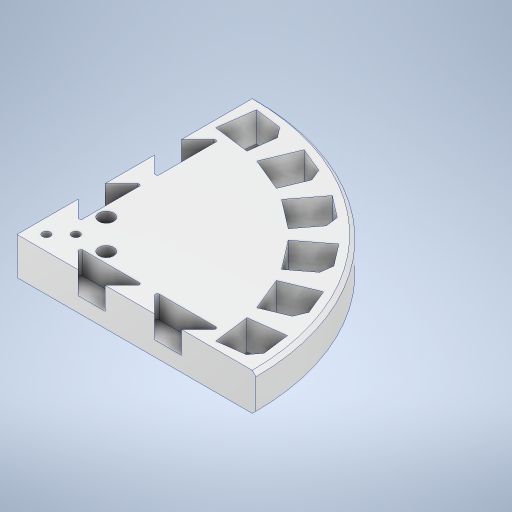
# Autodesk Inventor part: IPT_Quarter_Sample_Tray
Saved by Autodesk Inventor 2024 (Build 280153000, 153)
## iProperties
Created: 2023-10-26
Part Number: IPT_Quarter_Sample_Tray
Material: Generic
Document SubType Name: Modeling
Designer: Besher
Density: 1 g/cm^3
Appearance: Aluminum - Flat
Author: Besher
Autodesk Inventor part; units mm, degrees
ref_plane "YZ Plane" through (0, 0, 0) normal (1, 0, 0) x (0, 1, 0)
ref_plane "XZ Plane" through (0, 0, 0) normal (0, 1, 0) x (-1, 0, 0)
sketch "Sketch1" plane through (0, 0, 0) normal (0, 1, 0) x (-1, 0, 0)
  circle A0 centre (0, 0) radius 203.2
  dimension "d0" = 406.4
  constraints: 1 centre point
  measures "d0" diameter of A0
extrude "Extrusion1" add sketch "Sketch1" along normal blind 38.1
sketch "Sketch3" plane through (0, 38.1, 0) normal (0, 1, 0) x (1, 0, 0)
  circle A0 centre (0, 0) radius 203.2 projected
  line L0 (0, 203.2) -> (0, 177.8)
  line L1 (-15.367, 193.167) -> (15.367, 193.167)
  line L2 (15.367, 193.167) -> (15.367, 162.433)
  line L3 (15.367, 162.433) -> (-15.367, 162.433)
  line L4 (-15.367, 162.433) -> (-15.367, 193.167)
  line L5 (-15.367, 193.167) -> (15.367, 162.433) construction
  line L6 (15.367, 193.167) -> (-15.367, 162.433) construction
  dimension "d14" = 25.4
  dimension "d15" = 30.734
  dimension "d16" = 30.734
  constraints: 14 end point, 2 midpoint, 2 parallel, 1 horizontal, 1 perpendicular, 1 vertical, 1 vertical alignment, 1 other
  measures "d14" distance of L0.start L0.end
  measures "d15" distance of L2.end L3.end
  measures "d16" distance of L1.end L2.end
extrude "Extrusion2" cut sketch "Sketch3" against normal blind 25.4 contours L1 L2 L3 L4
sketch "Sketch4" plane through (0, 12.7, 0) normal (0, 1, 0) x (1, 0, 0)
  line L0 (15.367, 193.167) -> (15.367, 162.433) projected
  line L1 (15.367, 193.167) -> (7.747, 193.167)
  line L2 (-15.367, 193.167) -> (15.367, 193.167) projected
  line L3 (15.367, 193.167) -> (15.367, 185.547)
  line L4 (15.367, 185.547) -> (7.747, 193.167)
  point P0 (0, 0)
  dimension "d19" = 7.62
  dimension "d20" = 7.62
  constraints: 6 end point, 2 point on line
  measures "d19" distance of L0.start L1.end
  measures "d20" distance of L0.start L3.end
extrude "Extrusion3" add sketch "Sketch4" along normal up to surface (25.4 mm away)
pattern_circular "Circular Pattern1" count 24 over 360 about axis through (0, 0, 0) along (0, 1, 0) of "Extrusion2", "Extrusion3"
sketch "Sketch7" plane through (0, 0, 0) normal (0, 0, 1) x (1, 0, 0)
  line L0 (203.2, 0) -> (-203.2, 0) projected
  line L1 (-203.2, 0) -> (-203.2, 38.1) projected
  line L2 (203.2, 0) -> (-203.2, 0)
  line L3 (-203.2, 0) -> (-203.2, 6.35)
  line L4 (-203.2, 6.35) -> (203.2, 6.35)
  line L5 (203.2, 6.35) -> (203.2, 0)
  point P0 (0, 0)
  dimension "d49" = 6.35
  constraints: 8 end point, 2 parallel, 1 horizontal, 1 perpendicular, 1 point on line
  measures "d49" distance between parallel lines of L0 L4
extrude "Extrusion5" cut sketch "Sketch7" along normal through all both and the other way through all
sketch "Sketch15" plane through (0, 38.1, 0) normal (0, 1, 0) x (1, 0, 0)
  circle A0 centre (0, 0) radius 203.2 projected
  line L0 (62.8665, 175.2474) -> (57.4783, 184.5799) projected
  line L1 (57.4783, 184.5799) -> (35.1519, 190.5623) projected
  line L2 (35.1519, 190.5623) -> (27.1974, 160.8755) projected
  line L3 (27.1974, 160.8755) -> (56.8841, 152.921) projected
  line L4 (56.8841, 152.921) -> (62.8665, 175.2474) projected
  line L5 (106.0817, 153.0049) -> (103.2926, 163.414) projected
  line L6 (103.2926, 163.414) -> (83.2753, 174.971) projected
  line L7 (83.2753, 174.971) -> (67.9083, 148.3546) projected
  line L8 (67.9083, 148.3546) -> (94.5247, 132.9876) projected
  line L9 (94.5247, 132.9876) -> (106.0817, 153.0049) projected
  line L10 (142.0677, 120.3354) -> (142.0677, 131.1117) projected
  line L11 (142.0677, 131.1117) -> (125.7236, 147.4558) projected
  line L12 (125.7236, 147.4558) -> (103.9914, 125.7236) projected
  line L13 (103.9914, 125.7236) -> (125.7236, 103.9914) projected
  line L14 (125.7236, 103.9914) -> (142.0677, 120.3354) projected
  line L15 (168.3719, 79.4653) -> (171.161, 89.8744) projected
  line L16 (171.161, 89.8744) -> (159.604, 109.8917) projected
  line L17 (159.604, 109.8917) -> (132.9876, 94.5247) projected
  line L18 (132.9876, 94.5247) -> (148.3546, 67.9083) projected
  line L19 (148.3546, 67.9083) -> (168.3719, 79.4653) projected
  line L20 (183.2019, 33.1797) -> (188.5901, 42.5123) projected
  line L21 (188.5901, 42.5123) -> (182.6077, 64.8387) projected
  line L22 (182.6077, 64.8387) -> (152.921, 56.8841) projected
  line L23 (152.921, 56.8841) -> (160.8755, 27.1974) projected
  line L24 (160.8755, 27.1974) -> (183.2019, 33.1797) projected
  line L25 (185.547, -15.367) -> (193.167, -7.747) projected
  line L26 (193.167, -7.747) -> (193.167, 15.367) projected
  line L27 (193.167, 15.367) -> (162.433, 15.367) projected
  line L28 (162.433, 15.367) -> (162.433, -15.367) projected
  line L29 (162.433, -15.367) -> (185.547, -15.367) projected
  line L30 (175.2474, -62.8665) -> (184.5799, -57.4783) projected
  line L31 (184.5799, -57.4783) -> (190.5623, -35.1519) projected
  line L32 (190.5623, -35.1519) -> (160.8755, -27.1974) projected
  line L33 (160.8755, -27.1974) -> (152.921, -56.8841) projected
  line L34 (152.921, -56.8841) -> (175.2474, -62.8665) projected
  line L35 (153.0049, -106.0817) -> (163.414, -103.2926) projected
  line L36 (163.414, -103.2926) -> (174.971, -83.2753) projected
  line L37 (174.971, -83.2753) -> (148.3546, -67.9083) projected
  line L38 (148.3546, -67.9083) -> (132.9876, -94.5247) projected
  line L39 (132.9876, -94.5247) -> (153.0049, -106.0817) projected
  line L40 (120.3354, -142.0677) -> (131.1117, -142.0677) projected
  line L41 (131.1117, -142.0677) -> (147.4558, -125.7236) projected
  line L42 (147.4558, -125.7236) -> (125.7236, -103.9914) projected
  line L43 (125.7236, -103.9914) -> (103.9914, -125.7236) projected
  line L44 (103.9914, -125.7236) -> (120.3354, -142.0677) projected
  line L45 (79.4653, -168.3719) -> (89.8744, -171.161) projected
  line L46 (89.8744, -171.161) -> (109.8917, -159.604) projected
  line L47 (109.8917, -159.604) -> (94.5247, -132.9876) projected
  line L48 (94.5247, -132.9876) -> (67.9083, -148.3546) projected
  line L49 (67.9083, -148.3546) -> (79.4653, -168.3719) projected
  line L50 (33.1797, -183.2019) -> (42.5123, -188.5901) projected
  line L51 (42.5123, -188.5901) -> (64.8387, -182.6077) projected
  line L52 (64.8387, -182.6077) -> (56.8841, -152.921) projected
  line L53 (56.8841, -152.921) -> (27.1974, -160.8755) projected
  line L54 (27.1974, -160.8755) -> (33.1797, -183.2019) projected
  line L55 (-15.367, -185.547) -> (-7.747, -193.167) projected
  line L56 (-7.747, -193.167) -> (15.367, -193.167) projected
  line L57 (15.367, -193.167) -> (15.367, -162.433) projected
  line L58 (15.367, -162.433) -> (-15.367, -162.433) projected
  line L59 (-15.367, -162.433) -> (-15.367, -185.547) projected
  line L60 (-62.8665, -175.2474) -> (-57.4783, -184.5799) projected
  line L61 (-57.4783, -184.5799) -> (-35.1519, -190.5623) projected
  line L62 (-35.1519, -190.5623) -> (-27.1974, -160.8755) projected
  line L63 (-27.1974, -160.8755) -> (-56.8841, -152.921) projected
  line L64 (-56.8841, -152.921) -> (-62.8665, -175.2474) projected
  line L65 (-106.0817, -153.0049) -> (-103.2926, -163.414) projected
  line L66 (-103.2926, -163.414) -> (-83.2753, -174.971) projected
  line L67 (-83.2753, -174.971) -> (-67.9083, -148.3546) projected
  line L68 (-67.9083, -148.3546) -> (-94.5247, -132.9876) projected
  line L69 (-94.5247, -132.9876) -> (-106.0817, -153.0049) projected
  line L70 (-142.0677, -120.3354) -> (-142.0677, -131.1117) projected
  line L71 (-142.0677, -131.1117) -> (-125.7236, -147.4558) projected
  line L72 (-125.7236, -147.4558) -> (-103.9914, -125.7236) projected
  line L73 (-103.9914, -125.7236) -> (-125.7236, -103.9914) projected
  line L74 (-125.7236, -103.9914) -> (-142.0677, -120.3354) projected
  line L75 (-168.3719, -79.4653) -> (-171.161, -89.8744) projected
  line L76 (-171.161, -89.8744) -> (-159.604, -109.8917) projected
  line L77 (-159.604, -109.8917) -> (-132.9876, -94.5247) projected
  line L78 (-132.9876, -94.5247) -> (-148.3546, -67.9083) projected
  line L79 (-148.3546, -67.9083) -> (-168.3719, -79.4653) projected
  line L80 (-183.2019, -33.1797) -> (-188.5901, -42.5123) projected
  line L81 (-188.5901, -42.5123) -> (-182.6077, -64.8387) projected
  line L82 (-182.6077, -64.8387) -> (-152.921, -56.8841) projected
  line L83 (-152.921, -56.8841) -> (-160.8755, -27.1974) projected
  line L84 (-160.8755, -27.1974) -> (-183.2019, -33.1797) projected
  line L85 (-185.547, 15.367) -> (-193.167, 7.747) projected
  line L86 (-193.167, 7.747) -> (-193.167, -15.367) projected
  line L87 (-193.167, -15.367) -> (-162.433, -15.367) projected
  line L88 (-162.433, -15.367) -> (-162.433, 15.367) projected
  line L89 (-162.433, 15.367) -> (-185.547, 15.367) projected
  line L90 (-175.2474, 62.8665) -> (-184.5799, 57.4783) projected
  line L91 (-184.5799, 57.4783) -> (-190.5623, 35.1519) projected
  line L92 (-190.5623, 35.1519) -> (-160.8755, 27.1974) projected
  line L93 (-160.8755, 27.1974) -> (-152.921, 56.8841) projected
  line L94 (-152.921, 56.8841) -> (-175.2474, 62.8665) projected
  line L95 (-153.0049, 106.0817) -> (-163.414, 103.2926) projected
  line L96 (-163.414, 103.2926) -> (-174.971, 83.2753) projected
  line L97 (-174.971, 83.2753) -> (-148.3546, 67.9083) projected
  line L98 (-148.3546, 67.9083) -> (-132.9876, 94.5247) projected
  line L99 (-132.9876, 94.5247) -> (-153.0049, 106.0817) projected
  line L100 (-120.3354, 142.0677) -> (-131.1117, 142.0677) projected
  line L101 (-131.1117, 142.0677) -> (-147.4558, 125.7236) projected
  line L102 (-147.4558, 125.7236) -> (-125.7236, 103.9914) projected
  line L103 (-125.7236, 103.9914) -> (-103.9914, 125.7236) projected
  line L104 (-103.9914, 125.7236) -> (-120.3354, 142.0677) projected
  line L105 (-79.4653, 168.3719) -> (-89.8744, 171.161) projected
  line L106 (-89.8744, 171.161) -> (-109.8917, 159.604) projected
  line L107 (-109.8917, 159.604) -> (-94.5247, 132.9876) projected
  line L108 (-94.5247, 132.9876) -> (-67.9083, 148.3546) projected
  line L109 (-67.9083, 148.3546) -> (-79.4653, 168.3719) projected
  line L110 (-33.1797, 183.2019) -> (-42.5123, 188.5901) projected
  line L111 (-42.5123, 188.5901) -> (-64.8387, 182.6077) projected
  line L112 (-64.8387, 182.6077) -> (-56.8841, 152.921) projected
  line L113 (-56.8841, 152.921) -> (-27.1974, 160.8755) projected
  line L114 (-27.1974, 160.8755) -> (-33.1797, 183.2019) projected
  line L115 (15.367, 185.547) -> (7.747, 193.167) projected
  line L116 (7.747, 193.167) -> (-15.367, 193.167) projected
  line L117 (-15.367, 193.167) -> (-15.367, 162.433) projected
  line L118 (-15.367, 162.433) -> (15.367, 162.433) projected
  line L119 (15.367, 162.433) -> (15.367, 185.547) projected
  circle A1 centre (0, 0) radius 203.2 projected
  line L120 (-67.9083, 148.3546) -> (-56.8841, 152.921)
  line L121 (0, 0) -> (-77.7613, 187.7323)
  line L122 (0, 0) -> (187.7323, 77.7613)
  point P0 (-77.7613, 187.7323)
  point P1 (187.7323, 77.7613)
  constraints: 6 end point, 2 perpendicular, 2 point on circle
extrude "Extrusion7" cut sketch "Sketch15" against normal through all contours A0 L121 L122 | L24 L23 L22 L21 L20 | L29 L28 L27 L26 L25 | L34 L33 L32 L31 L30 | L39 L38 L37 L36 L35 | L44 L43 L42 L41 L40 | L49 L48 L47 L46 L45 | L54 L53 L52 L51 L50 | L59 L58 L57 L56 L55 | L64 L63 L62 L61 L60 | L69 L68 L67 L66 L65 | L74 L73 L72 L71 L70 | L79 L78 L77 L76 L75 | L84 L83 L82 L81 L80 | L89 L88 L87 L86 L85 | L94 L93 L92 L91 L90 | L99 L98 L97 L96 L95 | L104 L103 L102 L101 L100 | L109 L108 L107 L106 L105 picked at (0, -108.2887)
ref_plane "Work Plane1" through (187.7323, 6.35, -77.7613) normal (0.3826834, 0, 0.9238795) x (0.9238795, 0, -0.3826834)
move or copy body "Move Body1" bodies to move or copy 1 copy no rotation origin (0, 0, 0) rotation axis (0, 1, 0) rotation angle -22.5
move or copy body "Move Body2" bodies to move or copy 1 copy no translate (25.4, 0, 0)
sketch "Sketch28" plane through (25.4, 38.1, 0) normal (0, 1, 0) x (1, 0, 0)
  arc A0 (203.2, 0) -> (0, 203.2) centre (0, 0) ccw projected
  line L0 (-1.5825, 163.0492) -> (155.575, 163.0492)
  line L1 (1.8852, 28.7744) -> (217.4875, 28.7744)
  line L2 (42.8625, 163.0492) -> (42.8625, 28.7744)
  line L3 (42.8625, 95.9118) -> (-1.6357, 95.9118)
  line L4 (0, 117.0033) -> (0, 139.822)
  line L5 (0, 139.822) -> (13.8037, 153.6257)
  line L6 (16.5354, 152.4942) -> (16.5354, 104.3311)
  line L7 (13.8037, 103.1996) -> (0, 117.0033)
  arc A1 (16.5354, 152.4942) -> (13.8037, 153.6257) centre (14.9352, 152.4942) ccw
  arc A2 (13.8037, 103.1996) -> (16.5354, 104.3311) centre (14.9352, 104.3311) ccw
  line L8 (0, 139.822) -> (0, 163.0492) construction
  line L9 (0, 74.8202) -> (0, 52.0015)
  line L10 (0, 52.0015) -> (13.8037, 38.1978)
  line L11 (16.5354, 39.3293) -> (16.5354, 87.4924)
  line L12 (13.8037, 88.6239) -> (0, 74.8202)
  arc A3 (13.8037, 38.1978) -> (16.5354, 39.3293) centre (14.9352, 39.3293) ccw
  arc A4 (16.5354, 87.4924) -> (13.8037, 88.6239) centre (14.9352, 87.4924) ccw
  line L13 (0, 52.0015) -> (0, 28.7744) construction
  line L14 (0, 0) -> (143.6841, 143.6841)
  line L15 (117.0033, 0) -> (139.822, 0)
  line L16 (139.822, 0) -> (153.6257, 13.8037)
  line L17 (152.4942, 16.5354) -> (104.3311, 16.5354)
  line L18 (103.1996, 13.8037) -> (117.0033, 0)
  arc A5 (153.6257, 13.8037) -> (152.4942, 16.5354) centre (152.4942, 14.9352) ccw
  arc A6 (104.3311, 16.5354) -> (103.1996, 13.8037) centre (104.3311, 14.9352) ccw
  line L19 (139.822, 0) -> (163.0492, 0) construction
  line L20 (88.6239, 13.8037) -> (74.8202, 0)
  line L21 (74.8202, 0) -> (52.0015, 0)
  line L22 (39.3293, 16.5354) -> (87.4924, 16.5354)
  arc A7 (39.3293, 16.5354) -> (38.1978, 13.8037) centre (39.3293, 14.9352) ccw
  line L23 (52.0015, 0) -> (38.1978, 13.8037)
  line L24 (52.0015, 0) -> (28.7744, 0) construction
  arc A8 (88.6239, 13.8037) -> (87.4924, 16.5354) centre (87.4924, 14.9352) ccw
  point P0 (-25.4, 0)
  dimension "d126" = 1.6002
  dimension "d127" = 45
  dimension "d128" = 16.5354
  constraints: 50 end point, 27 symmetric about line, 17 point on circle, 8 centre point, 4 tangent, 3 horizontal, 3 perpendicular, 3 point on line, 1 equal radius, 1 midpoint, 1 parallel, 6 other
  measures "d126" radius of A1
  measures "d127" angle of L5 L6
  measures "d128" distance between parallel lines of L6 L4
extrude "Extrusion12" cut sketch "Sketch28" against normal blind 19.05 contours L4 L5 A1 L6 A2 L7 | L12 A4 L11 A3 L10 L9 | L18 A6 L17 A5 L16 L15 | L20 L21 L23 A7 L22 A8
sketch "Sketch31" plane through (165.222, 38.1, 0) normal (0, 1, 0) x (1, 0, 0)
  line L0 (-139.822, 52.0015) -> (-139.822, 0) construction
  line L1 (-139.822, 0) -> (-139.822, 244.475) construction
  line L2 (63.378, 0) -> (-139.822, 0) construction
  line L3 (-139.822, 0) -> (80.9625, 0) construction
  circle A0 centre (-261.42, 54.9858) radius 2.5
  circle A1 centre (-273.92, 67.4858) radius 2.5
  circle A2 centre (-261.42, 29.9858) radius 2.5
  circle A3 centre (-273.92, 17.4858) radius 2.5
  circle A4 centre (-223.92, 17.4858) radius 2.5
  circle A5 centre (-236.42, 29.9858) radius 2.5
  circle A6 centre (-127.322, 12.5) radius 3.3782
  circle A7 centre (-223.92, 67.4858) radius 2.5
  circle A8 centre (-248.92, 42.4858) radius 2.5
  circle A9 centre (-139.822, 0) radius 2.5
  line L4 (-248.92, 42.4858) -> (-266.7, 42.4858) construction
  line L5 (-248.92, 42.4858) -> (-261.42, 54.9858) construction
  line L6 (-139.822, 0) -> (-127.322, 12.5) construction
  line L7 (-127.322, 12.5) -> (-114.822, 25) construction
  circle A10 centre (-114.822, 25) radius 3.3782
  dimension "d144" = 220.7845
  dimension "d157" = 17.6777
  dimension "d158" = 12.5
  dimension "d160" = 17.6777
  dimension "d161" = 5
  dimension "d162" = 6.7564
  dimension "d163" = 6.7564
  constraints: 12 end point, 11 centre point, 10 coincident, 1 collinear, 1 horizontal, 1 vertical
  measures "d144" distance from line of L3.end L0
  measures "d157" distance of A6.centre L6.start
  measures "d158" horizontal distance of A6.centre L6.start
  measures "d160" distance of L6.end L7.end
  measures "d161" diameter of A9
  measures "d162" diameter of A10
  measures "d163" diameter of A6
extrude "Extrusion13" cut sketch "Sketch31" against normal through all contours A6 | A10
sketch "Sketch32" plane through (165.222, 38.1, 0) normal (0, 1, 0) x (1, 0, 0)
  line L0 (-139.822, 52.0015) -> (-139.822, 0) construction
  line L1 (-139.822, 0) -> (-139.822, 31.75) construction
  line L2 (-139.822, 0) -> (-87.8205, 0) construction
  line L3 (-139.822, 0) -> (-122.2375, 0) construction
  circle A0 centre (-114.522, 50.6) radius 6.35
  circle A1 centre (-89.222, 25.3) radius 6.35
  point P0 (-230.1763, -16.3822)
  point P1 (-114.522, -50.6)
  dimension "d174" = 50.6
  dimension "d175" = 25.3
  dimension "d176" = 12.7
  dimension "d177" = 12.7
  dimension "d178" = 25.3
  dimension "d179" = 50.6
  constraints: 4 end point, 2 centre point, 2 point on line
  measures "d174" distance from line of L2 A0.centre
  measures "d175" distance from line of L0 A0.centre
  measures "d176" diameter of A0
  measures "d177" diameter of A1
  measures "d178" distance from line of L2 A1.centre
  measures "d179" distance from line of L0 A1.centre
extrude "Extrusion14" cut sketch "Sketch32" against normal through all
chamfer "Chamfer1" distance 3.175 angle 45 2 edges at (169.0841, 38.1, -143.6841) (169.0841, 6.35, -143.6841)
body "Solid1"
